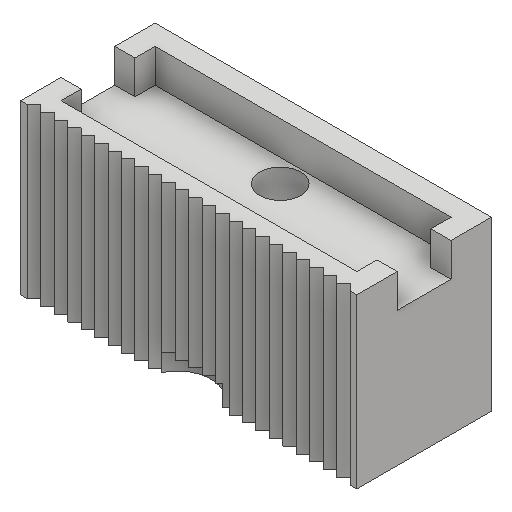
# Autodesk Inventor part: 3DP_ABS_Nozzle_Cleaner
Saved by Autodesk Inventor 2026.1 (Build 301233000, 233)
## iProperties
Created: 2016-06-28
Part Number: 3DP_ABS_Nozzle_Cleaner
Material: Ogólny
Document SubType Name: Modeling
Designer: Andrzej
Density: 1 g/cm^3
Appearance: Domyślna
Author: Andrzej
Autodesk Inventor part; units mm, degrees
ref_plane "YZ Plane" through (0, 0, 0) normal (1, 0, 0) x (0, 1, 0)
ref_plane "XZ Plane" through (0, 0, 0) normal (0, 1, 0) x (-1, 0, 0)
ref_plane "XY Plane" through (0, 0, 0) normal (0, 0, 1) x (1, 0, 0)
sketch "Szkic1" plane through (0, 0, 0) normal (0, 0, 1) x (1, 0, 0)
  line L0 (-6.3643, 3.3741) -> (43.6357, 3.3741)
  line L1 (43.6357, 3.3741) -> (43.6357, -16.6259)
  line L2 (43.6357, -16.6259) -> (-6.3643, -16.6259)
  line L3 (-6.3643, -16.6259) -> (-6.3643, 3.3741)
  point P0 (0, 0)
  dimension "d0" = 50
  dimension "d1" = 20
  constraints: 8 end point, 2 parallel, 1 horizontal, 1 perpendicular
  measures "d0" distance of L1.end L2.end
  measures "d1" distance of L0.end L1.end
extrude "Wyciągnięcie proste1" add sketch "Szkic1" along normal blind 20
sketch "Szkic2" plane through (0, 0, 20) normal (0, 0, 1) x (1, 0, 0)
  line L0 (43.6357, 3.3741) -> (-6.3643, 3.3741) projected
  line L1 (-6.3643, 3.3741) -> (-6.3643, -16.6259) projected
  line L2 (-6.3643, -16.6259) -> (43.6357, -16.6259) projected
  line L3 (43.6357, -16.6259) -> (43.6357, 3.3741) projected
  line L4 (-3.3643, 0.3741) -> (40.6357, 0.3741)
  line L5 (40.6357, -13.6259) -> (-3.3643, -13.6259)
  line L6 (-3.3643, -13.6259) -> (-3.3643, -10.6259)
  line L7 (-3.3643, -2.6259) -> (-3.3643, 0.3741)
  line L8 (-6.3643, -2.6259) -> (-3.3643, -2.6259)
  line L9 (40.6357, -2.6259) -> (43.6357, -2.6259)
  line L10 (-6.3643, -10.6259) -> (-3.3643, -10.6259)
  line L11 (40.6357, -10.6259) -> (43.6357, -10.6259)
  line L12 (40.6357, 0.3741) -> (40.6357, -2.6259)
  line L13 (40.6357, -10.6259) -> (40.6357, -13.6259)
  point P0 (0, 0)
  dimension "d4" = 3
  dimension "d7" = 6
  dimension "d8" = 6
  dimension "d9" = 6
  dimension "d10" = 6
  dimension "d11" = 3
  dimension "d12" = 3
  dimension "d13" = 3
  dimension "d14" = 3
  constraints: 20 end point, 4 horizontal, 4 point on line
  measures "d4" distance between parallel lines of L0 L4
  measures "d7" distance between parallel lines of L0 L8
  measures "d8" distance between parallel lines of L2 L10
  measures "d9" distance between parallel lines of L2 L11
  measures "d10" distance between parallel lines of L0 L9
  measures "d11" distance between parallel lines of L1 L7
  measures "d12" distance between parallel lines of L1 L6
  measures "d13" distance between parallel lines of L3 L13
  measures "d14" distance between parallel lines of L3 L12
extrude "Wyciągnięcie proste2" add sketch "Szkic2" along normal blind 5 contours L3 L9 L12 L4 L7 L8 L1 L0 | L3 L2 L1 L10 L6 L5 L13 L11
sketch "Szkic3" plane through (0, 0, 25) normal (0, 0, 1) x (1, 0, 0)
  line L0 (-6.3643, -16.6259) -> (43.6357, -16.6259) projected
  line L1 (43.6357, -16.6259) -> (43.6357, -10.6259) projected
  line L2 (43.6357, -10.6259) -> (40.6357, -10.6259) projected
  line L3 (40.6357, -10.6259) -> (40.6357, -13.6259) projected
  line L4 (40.6357, -13.6259) -> (-3.3643, -13.6259) projected
  line L5 (-3.3643, -13.6259) -> (-3.3643, -10.6259) projected
  line L6 (-3.3643, -10.6259) -> (-6.3643, -10.6259) projected
  line L7 (-6.3643, -10.6259) -> (-6.3643, -16.6259) projected
  line L8 (-6.3643, -16.6259) -> (43.6357, -16.6259) projected
  line L9 (-5.3643, -16.6259) -> (-3.3643, -16.6259)
  line L10 (-5.3643, -16.6259) -> (-4.3643, -15.6259)
  line L11 (-4.3643, -15.6259) -> (-3.3643, -16.6259)
  point P0 (0, 0)
  dimension "d17" = 2
  dimension "d18" = 1
  dimension "d19" = 1
  constraints: 6 end point, 2 point on line, 1 perpendicular
  measures "d17" distance of L9.start L9.end
  measures "d18" distance from line of L0 L10.end
  measures "d19" distance of L0.start L9.start
extrude "Wyciągnięcie proste3" cut sketch "Szkic3" against normal through all contours L10 L11 L0
pattern_linear "Szyk prostokątny1" count 24 spacing 2 along (1, 0, 0) of "Wyciągnięcie proste3"
sketch "Szkic4" plane through (0, 0, 0) normal (0, 0, -1) x (-1, 0, 0)
  line L0 (-42.6357, -16.6259) -> (-41.6357, -15.6259) projected
  line L1 (-41.6357, -15.6259) -> (-40.6357, -16.6259) projected
  line L2 (-40.6357, -16.6259) -> (-39.6357, -15.6259) projected
  line L3 (-39.6357, -15.6259) -> (-38.6357, -16.6259) projected
  line L4 (-38.6357, -16.6259) -> (-37.6357, -15.6259) projected
  line L5 (-37.6357, -15.6259) -> (-36.6357, -16.6259) projected
  line L6 (-36.6357, -16.6259) -> (-35.6357, -15.6259) projected
  line L7 (-35.6357, -15.6259) -> (-34.6357, -16.6259) projected
  line L8 (-34.6357, -16.6259) -> (-33.6357, -15.6259) projected
  line L9 (-33.6357, -15.6259) -> (-32.6357, -16.6259) projected
  line L10 (-32.6357, -16.6259) -> (-31.6357, -15.6259) projected
  line L11 (-31.6357, -15.6259) -> (-30.6357, -16.6259) projected
  line L12 (-30.6357, -16.6259) -> (-29.6357, -15.6259) projected
  line L13 (-29.6357, -15.6259) -> (-28.6357, -16.6259) projected
  line L14 (-28.6357, -16.6259) -> (-27.6357, -15.6259) projected
  line L15 (-27.6357, -15.6259) -> (-26.6357, -16.6259) projected
  line L16 (-26.6357, -16.6259) -> (-25.6357, -15.6259) projected
  line L17 (-25.6357, -15.6259) -> (-24.6357, -16.6259) projected
  line L18 (-24.6357, -16.6259) -> (-23.6357, -15.6259) projected
  line L19 (-23.6357, -15.6259) -> (-22.6357, -16.6259) projected
  line L20 (-22.6357, -16.6259) -> (-21.6357, -15.6259) projected
  line L21 (-21.6357, -15.6259) -> (-20.6357, -16.6259) projected
  line L22 (-20.6357, -16.6259) -> (-19.6357, -15.6259) projected
  line L23 (-19.6357, -15.6259) -> (-18.6357, -16.6259) projected
  line L24 (-18.6357, -16.6259) -> (-17.6357, -15.6259) projected
  line L25 (-17.6357, -15.6259) -> (-16.6357, -16.6259) projected
  line L26 (-16.6357, -16.6259) -> (-15.6357, -15.6259) projected
  line L27 (-15.6357, -15.6259) -> (-14.6357, -16.6259) projected
  line L28 (-14.6357, -16.6259) -> (-13.6357, -15.6259) projected
  line L29 (-13.6357, -15.6259) -> (-12.6357, -16.6259) projected
  line L30 (-12.6357, -16.6259) -> (-11.6357, -15.6259) projected
  line L31 (-11.6357, -15.6259) -> (-10.6357, -16.6259) projected
  line L32 (-10.6357, -16.6259) -> (-9.6357, -15.6259) projected
  line L33 (-9.6357, -15.6259) -> (-8.6357, -16.6259) projected
  line L34 (-8.6357, -16.6259) -> (-7.6357, -15.6259) projected
  line L35 (-7.6357, -15.6259) -> (-6.6357, -16.6259) projected
  line L36 (-6.6357, -16.6259) -> (-5.6357, -15.6259) projected
  line L37 (-5.6357, -15.6259) -> (-4.6357, -16.6259) projected
  line L38 (-4.6357, -16.6259) -> (-3.6357, -15.6259) projected
  line L39 (-3.6357, -15.6259) -> (-2.6357, -16.6259) projected
  line L40 (-2.6357, -16.6259) -> (-1.6357, -15.6259) projected
  line L41 (-1.6357, -15.6259) -> (-0.6357, -16.6259) projected
  line L42 (-0.6357, -16.6259) -> (0.3643, -15.6259) projected
  line L43 (0.3643, -15.6259) -> (1.3643, -16.6259) projected
  line L44 (1.3643, -16.6259) -> (2.3643, -15.6259) projected
  line L45 (2.3643, -15.6259) -> (3.3643, -16.6259) projected
  line L46 (3.3643, -16.6259) -> (4.3643, -15.6259) projected
  line L47 (4.3643, -15.6259) -> (5.3643, -16.6259) projected
  line L48 (5.3643, -16.6259) -> (6.3643, -16.6259) projected
  line L49 (6.3643, -16.6259) -> (6.3643, 3.3741) projected
  line L50 (6.3643, 3.3741) -> (-43.6357, 3.3741) projected
  line L51 (-43.6357, 3.3741) -> (-43.6357, -16.6259) projected
  line L52 (-43.6357, -16.6259) -> (-42.6357, -16.6259) projected
  circle A0 centre (-18.6357, -18.3259) radius 5
  point P0 (0, 0)
  point P1 (-18.6357, -3.0259)
  dimension "d25" = 25
  dimension "d26" = 6.4
  dimension "d27" = 10
  dimension "d28" = 15.3
  dimension "d29" = 25
  constraints: 1 centre point
  measures "d25" distance from line of L51 point (-18.636, -3.026)
  measures "d26" distance from line of point (-18.636, -3.026) L50
  measures "d27" diameter of A0
  measures "d28" distance of point (-18.636, -3.026) A0.centre
  measures "d29" distance from line of L51 A0.centre
extrude "Wyciągnięcie proste4" cut sketch "Szkic4" against normal blind 3.1 contours A0 L28 L27 L26 L25 L24 L23 L22 L21 L20 L19 | L19 L20 L21 L22 L23 L24 L25 L26 L27 L28 A0
hole "Otwór1" at (18.6357, -3.0259, 0) direction (0, 0, 1) diameter 3 end through all
sketch "Szkic5" plane through (0, 0, 20) normal (0, 0, 1) x (1, 0, 0)
  circle A0 centre (18.6357, -3.0259) radius 1.5 projected
  line L0 (-3.3643, -2.6259) -> (-6.3643, -2.6259) projected
  line L1 (-6.3643, -2.6259) -> (-6.3643, -10.6259) projected
  line L2 (-6.3643, -10.6259) -> (-3.3643, -10.6259) projected
  line L3 (-3.3643, -10.6259) -> (-3.3643, -13.6259) projected
  line L4 (-3.3643, -13.6259) -> (40.6357, -13.6259) projected
  line L5 (40.6357, -13.6259) -> (40.6357, -10.6259) projected
  line L6 (40.6357, -10.6259) -> (43.6357, -10.6259) projected
  line L7 (43.6357, -10.6259) -> (43.6357, -2.6259) projected
  line L8 (43.6357, -2.6259) -> (40.6357, -2.6259) projected
  line L9 (40.6357, -2.6259) -> (40.6357, 0.3741) projected
  line L10 (40.6357, 0.3741) -> (-3.3643, 0.3741) projected
  line L11 (-3.3643, 0.3741) -> (-3.3643, -2.6259) projected
  circle A1 centre (18.6357, -3.0259) radius 3.05
  point P0 (0, 0)
  dimension "d39" = 6.1
  constraints: 1 centre point, 1 coincident
  measures "d39" diameter of A1
extrude "Wyciągnięcie proste5" cut sketch "Szkic5" against normal blind 17 contours A1
